Autodesk Fusion 360 part; units mm, degrees
note: some values were not read from the file. Set by a fixed rule: which sketch regions a step uses.
(part 12 of 59)
  spline S64 degree 5 poles (17.8246, 37.863) (17.8224, 37.8615) (17.8179, 37.8584) (17.8112, 37.8539) (17.8023, 37.8477) (17.7913, 37.8401) (17.7802, 37.8325) (17.7692, 37.8248) (17.7583, 37.8172) (17.7473, 37.8096) (17.7364, 37.8019) (17.7256, 37.7943) (17.7147, 37.7867) (17.7039, 37.7791) (17.6932, 37.7715) (17.6825, 37.7639) (17.6718, 37.7563) (17.6611, 37.7487) (17.6505, 37.7411) (17.6399, 37.7335) (17.6294, 37.7259) (17.6189, 37.7184) (17.6084, 37.7108) (17.598, 37.7032) (17.5876, 37.6957) (17.5772, 37.6881) (17.5669, 37.6806) (17.5566, 37.6731) (17.5464, 37.6655) (17.5361, 37.658) (17.526, 37.6505) (17.5158, 37.643) (17.5057, 37.6355) (17.4956, 37.628) (17.4856, 37.6205) (17.4756, 37.613) (17.4657, 37.6055) (17.4557, 37.5981) (17.4458, 37.5906) (17.436, 37.5832) (17.4262, 37.5757) (17.4164, 37.5683) (17.4067, 37.5609) (17.397, 37.5534) (17.3873, 37.546) (17.3777, 37.5386) (17.3681, 37.5312) (17.3585, 37.5238) (17.349, 37.5165) (17.3395, 37.5091) (17.3301, 37.5017) (17.3207, 37.4944) (17.3113, 37.4871) (17.302, 37.4797) (17.2927, 37.4724) (17.2835, 37.4651) (17.2743, 37.4578) (17.2651, 37.4505) (17.2559, 37.4432) (17.2469, 37.436) (17.2378, 37.4287) (17.2288, 37.4215) (17.2198, 37.4142) (17.2108, 37.407) (17.2019, 37.3998) (17.1931, 37.3926) (17.1842, 37.3854) (17.1754, 37.3782) (17.1667, 37.3711) (17.158, 37.3639) (17.1493, 37.3568) (17.1407, 37.3496) (17.1321, 37.3425) (17.1235, 37.3354) (17.115, 37.3283) (17.1065, 37.3212) (17.0981, 37.3142) (17.0897, 37.3071) (17.0813, 37.3001) (17.073, 37.2931) (17.0647, 37.2861) (17.0565, 37.2791) (17.0483, 37.2721) (17.0401, 37.2651) (17.032, 37.2582) (17.0239, 37.2512) (17.0159, 37.2443) (17.0079, 37.2374) (16.9999, 37.2305) (16.992, 37.2236) (16.9841, 37.2168) (16.9763, 37.2099) (16.9685, 37.2031) (16.9607, 37.1963) (16.953, 37.1895) (16.9453, 37.1827) (16.9377, 37.1759) (16.9301, 37.1692) (16.9225, 37.1625) (16.915, 37.1558) (16.9075, 37.1491) (16.9001, 37.1424) (16.8927, 37.1357) (16.8854, 37.1291) (16.8781, 37.1225) (16.8708, 37.1159) (16.8636, 37.1093) (16.8564, 37.1027) (16.8492, 37.0962) (16.8421, 37.0897) (16.8351, 37.0831) (16.8281, 37.0767) (16.8211, 37.0702) (16.8142, 37.0638) (16.8073, 37.0573) (16.8004, 37.0509) (16.7936, 37.0446) (16.7869, 37.0382) (16.7801, 37.0319) (16.7735, 37.0255) (16.7668, 37.0192) (16.7602, 37.013) (16.7537, 37.0067) (16.7472, 37.0005) (16.7407, 36.9943) (16.7343, 36.9881) (16.7279, 36.982) (16.7216, 36.9758) (16.7153, 36.9697) (16.7091, 36.9636) (16.7029, 36.9576) (16.6967, 36.9515) (16.6906, 36.9455) (16.6845, 36.9395) (16.6785, 36.9336) (16.6725, 36.9277) (16.6666, 36.9218) (16.6607, 36.9159) (16.6549, 36.91) (16.6491, 36.9042) (16.6433, 36.8984) (16.6376, 36.8926) (16.6319, 36.8869) (16.6263, 36.8812) (16.6207, 36.8755) (16.6152, 36.8698) (16.6097, 36.8642) (16.6043, 36.8586) (16.5989, 36.853) (16.5935, 36.8475) (16.5882, 36.842) (16.583, 36.8365) (16.5778, 36.8311) (16.5726, 36.8257) (16.5675, 36.8203) (16.5624, 36.8149) (16.5574, 36.8096) (16.5524, 36.8043) (16.5475, 36.7991) (16.5426, 36.7939) (16.5378, 36.7887) (16.533, 36.7835) (16.5282, 36.7784) (16.5236, 36.7733) (16.5189, 36.7683) (16.5143, 36.7633) (16.5098, 36.7583) (16.5053, 36.7534) (16.5008, 36.7485) (16.4964, 36.7436) (16.492, 36.7388) (16.4877, 36.734) (16.4835, 36.7293) (16.4793, 36.7246) (16.4751, 36.7199) (16.471, 36.7153) (16.4669, 36.7107) (16.4629, 36.7062) (16.459, 36.7017) (16.455, 36.6972) (16.4512, 36.6928) (16.4474, 36.6884) (16.4436, 36.6841) (16.4399, 36.6798) (16.4362, 36.6755) (16.4326, 36.6713) (16.4291, 36.6672) (16.4256, 36.6631) (16.4221, 36.659) (16.4187, 36.655) (16.4153, 36.651) (16.412, 36.6471) (16.4088, 36.6432) (16.4056, 36.6394) (16.4024, 36.6356) (16.3994, 36.6319) (16.3963, 36.6283) (16.3933, 36.6246) (16.3904, 36.6211) (16.3875, 36.6176) (16.3847, 36.6141) (16.3819, 36.6107) (16.3792, 36.6073) (16.3766, 36.604) (16.374, 36.6008) (16.3714, 36.5976) (16.3689, 36.5945) (16.3665, 36.5914) (16.3641, 36.5884) (16.3618, 36.5855) (16.3595, 36.5826) (16.3573, 36.5798) (16.3551, 36.577) (16.353, 36.5743) (16.351, 36.5717) (16.349, 36.5691) (16.3471, 36.5666) (16.3452, 36.5641) (16.3434, 36.5618) (16.3416, 36.5595) (16.3399, 36.5572) (16.3383, 36.5551) (16.3367, 36.553) (16.3352, 36.551) (16.3338, 36.549) (16.3324, 36.5471) (16.331, 36.5453) (16.3298, 36.5436) (16.3286, 36.542) (16.3274, 36.5404) (16.3263, 36.5389) (16.3253, 36.5375) (16.3244, 36.5362) (16.3235, 36.535) (16.3227, 36.5338) (16.3219, 36.5327) (16.3212, 36.5317) (16.3206, 36.5309) (16.32, 36.5301) (16.3195, 36.5294) (16.3191, 36.5287) (16.3188, 36.5283) (16.3186, 36.5281) (16.3185, 36.5279) (16.3184, 36.5278) knots -1 -1 -1 -1 -1 -1 -0.99583333 -0.99166667 -0.9875 -0.98333333 -0.97916667 -0.975 -0.97083333 -0.96666667 -0.9625 -0.95833333 -0.95416667 -0.95 -0.94583333 -0.94166667 -0.9375 -0.93333333 -0.92916667 -0.925 -0.92083333 -0.91666667 -0.9125 -0.90833333 -0.90416667 -0.9 -0.89583333 -0.89166667 -0.8875 -0.88333333 -0.87916667 -0.875 -0.87083333 -0.86666667 -0.8625 -0.85833333 -0.85416667 -0.85 -0.84583333 -0.84166667 -0.8375 -0.83333333 -0.82916667 -0.825 -0.82083333 -0.81666667 -0.8125 -0.80833333 -0.80416667 -0.8 -0.79583333 -0.79166667 -0.7875 -0.78333333 -0.77916667 -0.775 -0.77083333 -0.76666667 -0.7625 -0.75833333 -0.75416667 -0.75 -0.74583333 -0.74166667 -0.7375 -0.73333333 -0.72916667 -0.725 -0.72083333 -0.71666667 -0.7125 -0.70833333 -0.70416667 -0.7 -0.69583333 -0.69166667 -0.6875 -0.68333333 -0.67916667 -0.675 -0.67083333 -0.66666667 -0.6625 -0.65833333 -0.65416667 -0.65 -0.64583333 -0.64166667 -0.6375 -0.63333333 -0.62916667 -0.625 -0.62083333 -0.61666667 -0.6125 -0.60833333 -0.60416667 -0.6 -0.59583333 -0.59166667 -0.5875 -0.58333333 -0.57916667 -0.575 -0.57083333 -0.56666667 -0.5625 -0.55833333 -0.55416667 -0.55 -0.54583333 -0.54166667 -0.5375 -0.53333333 -0.52916667 -0.525 -0.52083333 -0.51666667 -0.5125 -0.50833333 -0.50416667 -0.5 -0.49583333 -0.49166667 -0.4875 -0.48333333 -0.47916667 -0.475 -0.47083333 -0.46666667 -0.4625 -0.45833333 -0.45416667 -0.45 -0.44583333 -0.44166667 -0.4375 -0.43333333 -0.42916667 -0.425 -0.42083333 -0.41666667 -0.4125 -0.40833333 -0.40416667 -0.4 -0.39583333 -0.39166667 -0.3875 -0.38333333 -0.37916667 -0.375 -0.37083333 -0.36666667 -0.3625 -0.35833333 -0.35416667 -0.35 -0.34583333 -0.34166667 -0.3375 -0.33333333 -0.32916667 -0.325 -0.32083333 -0.31666667 -0.3125 -0.30833333 -0.30416667 -0.3 -0.29583333 -0.29166667 -0.2875 -0.28333333 -0.27916667 -0.275 -0.27083333 -0.26666667 -0.2625 -0.25833333 -0.25416667 -0.25 -0.24583333 -0.24166667 -0.2375 -0.23333333 -0.22916667 -0.225 -0.22083333 -0.21666667 -0.2125 -0.20833333 -0.20416667 -0.2 -0.19583333 -0.19166667 -0.1875 -0.18333333 -0.17916667 -0.175 -0.17083333 -0.16666667 -0.1625 -0.15833333 -0.15416667 -0.15 -0.14583333 -0.14166667 -0.1375 -0.13333333 -0.12916667 -0.125 -0.12083333 -0.11666667 -0.1125 -0.10833333 -0.10416667 -0.1 -0.09583333 -0.09166667 -0.0875 -0.08333333 -0.07916667 -0.075 -0.07083333 -0.06666667 -0.0625 -0.05833333 -0.05416667 -0.05 -0.04583333 -0.04166667 -0.0375 -0.03333333 -0.02916667 -0.025 -0.02083333 -0.01666667 -0.0125 -0.00833333 -0.00416667 0 0 0 0 0 0
  line L140 (26.8955, 1.5338) -> (26.8948, 1.5341)
  line L141 (12.6495, -13.6461) -> (12.6491, -13.6453)
  line L142 (-28.9671, 14.6182) -> (-28.6734, 14.5967)
  line L143 (20.9575, 32.61) -> (20.9569, 32.6094)
  line L144 (21.9649, 31.0501) -> (22.1898, 31.2401)
  line L145 (-28.2039, 5.5632) -> (-27.918, 5.6335)
  spline S65 degree 5 poles (18.7406, -9.6904) (18.7407, -9.6905) (18.7408, -9.6907) (18.741, -9.6909) (18.7414, -9.6913) (18.7419, -9.6919) (18.7424, -9.6925) (18.7431, -9.6933) (18.7438, -9.6941) (18.7446, -9.695) (18.7455, -9.696) (18.7464, -9.697) (18.7474, -9.6982) (18.7485, -9.6994) (18.7497, -9.7007) (18.7509, -9.702) (18.7522, -9.7035) (18.7536, -9.705) (18.755, -9.7066) (18.7565, -9.7082) (18.7581, -9.7099) (18.7597, -9.7117) (18.7615, -9.7136) (18.7632, -9.7155) (18.7651, -9.7175) (18.767, -9.7195) (18.769, -9.7216) (18.771, -9.7238) (18.7732, -9.726) (18.7753, -9.7283) (18.7776, -9.7307) (18.7799, -9.7331) (18.7823, -9.7355) (18.7847, -9.738) (18.7872, -9.7406) (18.7897, -9.7433) (18.7924, -9.7459) (18.7951, -9.7487) (18.7978, -9.7515) (18.8006, -9.7543) (18.8035, -9.7572) (18.8064, -9.7602) (18.8094, -9.7632) (18.8124, -9.7662) (18.8156, -9.7693) (18.8187, -9.7725) (18.822, -9.7757) (18.8252, -9.7789) (18.8286, -9.7822) (18.832, -9.7855) (18.8355, -9.7889) (18.839, -9.7923) (18.8426, -9.7958) (18.8462, -9.7993) (18.8499, -9.8029) (18.8536, -9.8065) (18.8574, -9.8101) (18.8613, -9.8138) (18.8652, -9.8175) (18.8692, -9.8212) (18.8732, -9.825) (18.8773, -9.8289) (18.8814, -9.8328) (18.8856, -9.8367) (18.8899, -9.8406) (18.8942, -9.8446) (18.8986, -9.8486) (18.903, -9.8527) (18.9074, -9.8568) (18.9119, -9.8609) (18.9165, -9.8651) (18.9211, -9.8693) (18.9258, -9.8736) (18.9306, -9.8778) (18.9353, -9.8821) (18.9402, -9.8865) (18.9451, -9.8909) (18.95, -9.8953) (18.955, -9.8997) (18.96, -9.9042) (18.9651, -9.9087) (18.9703, -9.9132) (18.9755, -9.9177) (18.9807, -9.9223) (18.986, -9.927) (18.9914, -9.9316) (18.9968, -9.9363) (19.0022, -9.941) (19.0077, -9.9457) (19.0133, -9.9505) (19.0189, -9.9553) (19.0246, -9.9601) (19.0303, -9.9649) (19.036, -9.9698) (19.0418, -9.9747) (19.0477, -9.9796) (19.0536, -9.9846) (19.0595, -9.9895) (19.0655, -9.9945) (19.0715, -9.9996) (19.0776, -10.0046) (19.0838, -10.0097) (19.09, -10.0148) (19.0962, -10.0199) (19.1025, -10.025) (19.1088, -10.0302) (19.1152, -10.0354) (19.1216, -10.0406) (19.1281, -10.0458) (19.1346, -10.0511) (19.1412, -10.0564) (19.1478, -10.0617) (19.1544, -10.067) (19.1611, -10.0723) (19.1679, -10.0777) (19.1747, -10.083) (19.1815, -10.0884) (19.1884, -10.0939) (19.1954, -10.0993) (19.2024, -10.1048) (19.2094, -10.1102) (19.2165, -10.1157) (19.2236, -10.1212) (19.2307, -10.1268) (19.2379, -10.1323) (19.2452, -10.1379) (19.2525, -10.1435) (19.2598, -10.1491) (19.2672, -10.1547) (19.2747, -10.1603) (19.2821, -10.166) (19.2897, -10.1716) (19.2972, -10.1773) (19.3048, -10.183) (19.3125, -10.1887) (19.3202, -10.1945) (19.3279, -10.2002) (19.3357, -10.206) (19.3436, -10.2118) (19.3514, -10.2175) (19.3593, -10.2233) (19.3673, -10.2292) (19.3753, -10.235) (19.3834, -10.2408) (19.3914, -10.2467) (19.3996, -10.2526) (19.4078, -10.2585) (19.416, -10.2644) (19.4242, -10.2703) (19.4325, -10.2762) (19.4409, -10.2822) (19.4493, -10.2881) (19.4577, -10.2941) (19.4662, -10.3) (19.4747, -10.306) (19.4832, -10.312) (19.4918, -10.318) (19.5005, -10.3241) (19.5091, -10.3301) (19.5179, -10.3361) (19.5266, -10.3422) (19.5354, -10.3483) (19.5443, -10.3543) (19.5532, -10.3604) (19.5621, -10.3665) (19.5711, -10.3726) (19.5801, -10.3787) (19.5891, -10.3849) (19.5982, -10.391) (19.6073, -10.3971) (19.6165, -10.4033) (19.6257, -10.4095) (19.635, -10.4156) (19.6443, -10.4218) (19.6536, -10.428) (19.663, -10.4342) (19.6724, -10.4404) (19.6818, -10.4466) (19.6913, -10.4528) (19.7009, -10.4591) (19.7104, -10.4653) (19.72, -10.4715) (19.7297, -10.4778) (19.7394, -10.484) (19.7491, -10.4903) (19.7589, -10.4966) (19.7687, -10.5029) (19.7785, -10.5091) (19.7884, -10.5154) (19.7984, -10.5217) (19.8083, -10.528) (19.8183, -10.5343) (19.8284, -10.5406) (19.8384, -10.547) (19.8486, -10.5533) (19.8587, -10.5596) (19.8689, -10.566) (19.8791, -10.5723) (19.8894, -10.5786) (19.8997, -10.585) (19.9101, -10.5914) (19.9205, -10.5977) (19.9309, -10.6041) (19.9413, -10.6104) (19.9518, -10.6168) (19.9624, -10.6232) (19.973, -10.6296) (19.9836, -10.636) (19.9942, -10.6423) (20.0049, -10.6487) (20.0156, -10.6551) (20.0264, -10.6615) (20.0372, -10.6679) (20.048, -10.6743) (20.0589, -10.6807) (20.0698, -10.6872) (20.0808, -10.6936) (20.0917, -10.7) (20.1028, -10.7064) (20.1138, -10.7128) (20.1249, -10.7193) (20.136, -10.7257) (20.1472, -10.7321) (20.1584, -10.7385) (20.1697, -10.745) (20.1809, -10.7514) (20.1922, -10.7578) (20.2036, -10.7643) (20.215, -10.7707) (20.2264, -10.7771) (20.2379, -10.7836) (20.2493, -10.79) (20.2609, -10.7965) (20.2724, -10.8029) (20.284, -10.8094) (20.2957, -10.8158) (20.3073, -10.8222) (20.319, -10.8287) (20.3308, -10.8351) (20.3426, -10.8416) (20.3544, -10.848) (20.3639, -10.8532) (20.371, -10.8571) (20.3757, -10.8596) (20.3781, -10.8609) knots 0 0 0 0 0 0 0.00416667 0.00833333 0.0125 0.01666667 0.02083333 0.025 0.02916667 0.03333333 0.0375 0.04166667 0.04583333 0.05 0.05416667 0.05833333 0.0625 0.06666667 0.07083333 0.075 0.07916667 0.08333333 0.0875 0.09166667 0.09583333 0.1 0.10416667 0.10833333 0.1125 0.11666667 0.12083333 0.125 0.12916667 0.13333333 0.1375 0.14166667 0.14583333 0.15 0.15416667 0.15833333 0.1625 0.16666667 0.17083333 0.175 0.17916667 0.18333333 0.1875 0.19166667 0.19583333 0.2 0.20416667 0.20833333 0.2125 0.21666667 0.22083333 0.225 0.22916667 0.23333333 0.2375 0.24166667 0.24583333 0.25 0.25416667 0.25833333 0.2625 0.26666667 0.27083333 0.275 0.27916667 0.28333333 0.2875 0.29166667 0.29583333 0.3 0.30416667 0.30833333 0.3125 0.31666667 0.32083333 0.325 0.32916667 0.33333333 0.3375 0.34166667 0.34583333 0.35 0.35416667 0.35833333 0.3625 0.36666667 0.37083333 0.375 0.37916667 0.38333333 0.3875 0.39166667 0.39583333 0.4 0.40416667 0.40833333 0.4125 0.41666667 0.42083333 0.425 0.42916667 0.43333333 0.4375 0.44166667 0.44583333 0.45 0.45416667 0.45833333 0.4625 0.46666667 0.47083333 0.475 0.47916667 0.48333333 0.4875 0.49166667 0.49583333 0.5 0.50416667 0.50833333 0.5125 0.51666667 0.52083333 0.525 0.52916667 0.53333333 0.5375 0.54166667 0.54583333 0.55 0.55416667 0.55833333 0.5625 0.56666667 0.57083333 0.575 0.57916667 0.58333333 0.5875 0.59166667 0.59583333 0.6 0.60416667 0.60833333 0.6125 0.61666667 0.62083333 0.625 0.62916667 0.63333333 0.6375 0.64166667 0.64583333 0.65 0.65416667 0.65833333 0.6625 0.66666667 0.67083333 0.675 0.67916667 0.68333333 0.6875 0.69166667 0.69583333 0.7 0.70416667 0.70833333 0.7125 0.71666667 0.72083333 0.725 0.72916667 0.73333333 0.7375 0.74166667 0.74583333 0.75 0.75416667 0.75833333 0.7625 0.76666667 0.77083333 0.775 0.77916667 0.78333333 0.7875 0.79166667 0.79583333 0.8 0.80416667 0.80833333 0.8125 0.81666667 0.82083333 0.825 0.82916667 0.83333333 0.8375 0.84166667 0.84583333 0.85 0.85416667 0.85833333 0.8625 0.86666667 0.87083333 0.875 0.87916667 0.88333333 0.8875 0.89166667 0.89583333 0.9 0.90416667 0.90833333 0.9125 0.91666667 0.92083333 0.925 0.92916667 0.93333333 0.9375 0.94166667 0.94583333 0.95 0.95416667 0.95833333 0.9625 0.96666667 0.97083333 0.975 0.97916667 0.98333333 0.9875 0.99166667 0.99583333 1 1 1 1 1 1
  arc A72 (-13.0527, -15.6181) -> (-12.1618, -16.0147) centre (0, 12.5) ccw
  arc A73 (-13.578, -12.8417) -> (-12.5209, -13.3803) centre (0, 12.5) ccw
  arc A74 (20.3781, -10.8609) -> (21.1029, -10.2084) centre (0, 12.5) ccw
  spline S66 degree 5 poles (-30.8773, 15.255) (-30.8749, 15.2539) (-30.87, 15.2515) (-30.8627, 15.248) (-30.853, 15.2434) (-30.8408, 15.2376) (-30.8287, 15.2319) (-30.8165, 15.2262) (-30.8044, 15.2205) (-30.7924, 15.2149) (-30.7803, 15.2092) (-30.7683, 15.2036) (-30.7563, 15.1981) (-30.7443, 15.1925) (-30.7323, 15.187) (-30.7204, 15.1815) (-30.7085, 15.1761) (-30.6966, 15.1707) (-30.6847, 15.1653) (-30.6728, 15.1599) (-30.661, 15.1545) (-30.6492, 15.1492) (-30.6374, 15.1439) (-30.6256, 15.1387) (-30.6139, 15.1335) (-30.6022, 15.1283) (-30.5905, 15.1231) (-30.5788, 15.1179) (-30.5672, 15.1128) (-30.5555, 15.1077) (-30.5439, 15.1027) (-30.5324, 15.0977) (-30.5208, 15.0927) (-30.5093, 15.0877) (-30.4978, 15.0827) (-30.4863, 15.0778) (-30.4749, 15.0729) (-30.4634, 15.0681) (-30.452, 15.0632) (-30.4407, 15.0584) (-30.4293, 15.0537) (-30.418, 15.0489) (-30.4067, 15.0442) (-30.3954, 15.0395) (-30.3841, 15.0348) (-30.3729, 15.0302) (-30.3617, 15.0256) (-30.3506, 15.021) (-30.3394, 15.0165) (-30.3283, 15.0119) (-30.3172, 15.0074) (-30.3061, 15.003) (-30.2951, 14.9985) (-30.2841, 14.9941) (-30.2731, 14.9897) (-30.2621, 14.9854) (-30.2512, 14.981) (-30.2403, 14.9767) (-30.2294, 14.9725) (-30.2186, 14.9682) (-30.2078, 14.964) (-30.197, 14.9598) (-30.1862, 14.9557) (-30.1755, 14.9515) (-30.1648, 14.9474) (-30.1541, 14.9433) (-30.1435, 14.9393) (-30.1329, 14.9353) (-30.1223, 14.9313) (-30.1118, 14.9273) (-30.1012, 14.9234) (-30.0907, 14.9194) (-30.0803, 14.9156) (-30.0699, 14.9117) (-30.0595, 14.9079) (-30.0491, 14.9041) (-30.0388, 14.9003) (-30.0284, 14.8965) (-30.0182, 14.8928) (-30.0079, 14.8891) (-29.9977, 14.8855) (-29.9875, 14.8818) (-29.9774, 14.8782) (-29.9673, 14.8746) (-29.9572, 14.8711) (-29.9471, 14.8675) (-29.9371, 14.864) (-29.9271, 14.8606) (-29.9172, 14.8571) (-29.9073, 14.8537) (-29.8974, 14.8503) (-29.8875, 14.8469) (-29.8777, 14.8436) (-29.868, 14.8403) (-29.8582, 14.837) (-29.8485, 14.8337) (-29.8388, 14.8305) (-29.8292, 14.8273) (-29.8196, 14.8241) (-29.81, 14.821) (-29.8005, 14.8178) (-29.791, 14.8147) (-29.7815, 14.8117) (-29.7721, 14.8086) (-29.7627, 14.8056) (-29.7534, 14.8026) (-29.7441, 14.7996) (-29.7348, 14.7967) (-29.7255, 14.7938) (-29.7163, 14.7909) (-29.7072, 14.788) (-29.6981, 14.7852) (-29.689, 14.7824) (-29.6799, 14.7796) (-29.6709, 14.7769) (-29.6619, 14.7741) (-29.653, 14.7714) (-29.6441, 14.7688) (-29.6353, 14.7661) (-29.6265, 14.7635) (-29.6177, 14.7609) (-29.609, 14.7583) (-29.6003, 14.7558) (-29.5917, 14.7533) (-29.583, 14.7508) (-29.5745, 14.7483) (-29.566, 14.7458) (-29.5575, 14.7434) (-29.5491, 14.741) (-29.5407, 14.7387) (-29.5323, 14.7363) (-29.524, 14.734) (-29.5158, 14.7317) (-29.5075, 14.7295) (-29.4994, 14.7272) (-29.4912, 14.725) (-29.4832, 14.7228) (-29.4751, 14.7207) (-29.4671, 14.7185) (-29.4592, 14.7164) (-29.4513, 14.7143) (-29.4434, 14.7123) (-29.4356, 14.7102) (-29.4279, 14.7082) (-29.4202, 14.7062) (-29.4125, 14.7043) (-29.4049, 14.7023) (-29.3973, 14.7004) (-29.3898, 14.6985) (-29.3823, 14.6967) (-29.3749, 14.6948) (-29.3675, 14.693) (-29.3602, 14.6912) (-29.3529, 14.6895) (-29.3457, 14.6877) (-29.3386, 14.686) (-29.3314, 14.6843) (-29.3244, 14.6827) (-29.3174, 14.681) (-29.3104, 14.6794) (-29.3035, 14.6778) (-29.2967, 14.6762) (-29.2899, 14.6747) (-29.2831, 14.6731) (-29.2764, 14.6716) (-29.2698, 14.6702) (-29.2632, 14.6687) (-29.2567, 14.6673) (-29.2502, 14.6659) (-29.2438, 14.6645) (-29.2374, 14.6631) (-29.2311, 14.6618) (-29.2249, 14.6605) (-29.2187, 14.6592) (-29.2126, 14.6579) (-29.2065, 14.6567) (-29.2005, 14.6554) (-29.1946, 14.6542) (-29.1887, 14.653) (-29.1829, 14.6519) (-29.1771, 14.6507) (-29.1714, 14.6496) (-29.1658, 14.6485) (-29.1602, 14.6475) (-29.1547, 14.6464) (-29.1493, 14.6454) (-29.1439, 14.6444) (-29.1386, 14.6434) (-29.1334, 14.6424) (-29.1282, 14.6415) (-29.1231, 14.6406) (-29.118, 14.6397) (-29.1131, 14.6388) (-29.1081, 14.638) (-29.1033, 14.6371) (-29.0985, 14.6363) (-29.0938, 14.6355) (-29.0892, 14.6347) (-29.0847, 14.634) (-29.0802, 14.6332) (-29.0758, 14.6325) (-29.0714, 14.6318) (-29.0672, 14.6312) (-29.063, 14.6305) (-29.0589, 14.6299) (-29.0549, 14.6292) (-29.0509, 14.6286) (-29.047, 14.6281) (-29.0432, 14.6275) (-29.0395, 14.627) (-29.0359, 14.6264) (-29.0323, 14.6259) (-29.0289, 14.6254) (-29.0255, 14.625) (-29.0222, 14.6245) (-29.0189, 14.6241) (-29.0158, 14.6237) (-29.0128, 14.6233) (-29.0098, 14.6229) (-29.0069, 14.6225) (-29.0041, 14.6222) (-29.0015, 14.6219) (-28.9989, 14.6215) (-28.9963, 14.6212) (-28.9939, 14.621) (-28.9916, 14.6207) (-28.9894, 14.6204) (-28.9873, 14.6202) (-28.9852, 14.62) (-28.9833, 14.6198) (-28.9815, 14.6196) (-28.9798, 14.6194) (-28.9781, 14.6192) (-28.9766, 14.6191) (-28.9752, 14.6189) (-28.9739, 14.6188) (-28.9727, 14.6187) (-28.9716, 14.6186) (-28.9706, 14.6185) (-28.9698, 14.6184) (-28.969, 14.6184) (-28.9685, 14.6183) (-28.9682, 14.6183) (-28.968, 14.6183) (-28.9679, 14.6183) knots -1 -1 -1 -1 -1 -1 -0.99583333 -0.99166667 -0.9875 -0.98333333 -0.97916667 -0.975 -0.97083333 -0.96666667 -0.9625 -0.95833333 -0.95416667 -0.95 -0.94583333 -0.94166667 -0.9375 -0.93333333 -0.92916667 -0.925 -0.92083333 -0.91666667 -0.9125 -0.90833333 -0.90416667 -0.9 -0.89583333 -0.89166667 -0.8875 -0.88333333 -0.87916667 -0.875 -0.87083333 -0.86666667 -0.8625 -0.85833333 -0.85416667 -0.85 -0.84583333 -0.84166667 -0.8375 -0.83333333 -0.82916667 -0.825 -0.82083333 -0.81666667 -0.8125 -0.80833333 -0.80416667 -0.8 -0.79583333 -0.79166667 -0.7875 -0.78333333 -0.77916667 -0.775 -0.77083333 -0.76666667 -0.7625 -0.75833333 -0.75416667 -0.75 -0.74583333 -0.74166667 -0.7375 -0.73333333 -0.72916667 -0.725 -0.72083333 -0.71666667 -0.7125 -0.70833333 -0.70416667 -0.7 -0.69583333 -0.69166667 -0.6875 -0.68333333 -0.67916667 -0.675 -0.67083333 -0.66666667 -0.6625 -0.65833333 -0.65416667 -0.65 -0.64583333 -0.64166667 -0.6375 -0.63333333 -0.62916667 -0.625 -0.62083333 -0.61666667 -0.6125 -0.60833333 -0.60416667 -0.6 -0.59583333 -0.59166667 -0.5875 -0.58333333 -0.57916667 -0.575 -0.57083333 -0.56666667 -0.5625 -0.55833333 -0.55416667 -0.55 -0.54583333 -0.54166667 -0.5375 -0.53333333 -0.52916667 -0.525 -0.52083333 -0.51666667 -0.5125 -0.50833333 -0.50416667 -0.5 -0.49583333 -0.49166667 -0.4875 -0.48333333 -0.47916667 -0.475 -0.47083333 -0.46666667 -0.4625 -0.45833333 -0.45416667 -0.45 -0.44583333 -0.44166667 -0.4375 -0.43333333 -0.42916667 -0.425 -0.42083333 -0.41666667 -0.4125 -0.40833333 -0.40416667 -0.4 -0.39583333 -0.39166667 -0.3875 -0.38333333 -0.37916667 -0.375 -0.37083333 -0.36666667 -0.3625 -0.35833333 -0.35416667 -0.35 -0.34583333 -0.34166667 -0.3375 -0.33333333 -0.32916667 -0.325 -0.32083333 -0.31666667 -0.3125 -0.30833333 -0.30416667 -0.3 -0.29583333 -0.29166667 -0.2875 -0.28333333 -0.27916667 -0.275 -0.27083333 -0.26666667 -0.2625 -0.25833333 -0.25416667 -0.25 -0.24583333 -0.24166667 -0.2375 -0.23333333 -0.22916667 -0.225 -0.22083333 -0.21666667 -0.2125 -0.20833333 -0.20416667 -0.2 -0.19583333 -0.19166667 -0.1875 -0.18333333 -0.17916667 -0.175 -0.17083333 -0.16666667 -0.1625 -0.15833333 -0.15416667 -0.15 -0.14583333 -0.14166667 -0.1375 -0.13333333 -0.12916667 -0.125 -0.12083333 -0.11666667 -0.1125 -0.10833333 -0.10416667 -0.1 -0.09583333 -0.09166667 -0.0875 -0.08333333 -0.07916667 -0.075 -0.07083333 -0.06666667 -0.0625 -0.05833333 -0.05416667 -0.05 -0.04583333 -0.04166667 -0.0375 -0.03333333 -0.02916667 -0.025 -0.02083333 -0.01666667 -0.0125 -0.00833333 -0.00416667 0 0 0 0 0 0
  line L146 (22.9448, 30.3091) -> (22.9441, 30.3086)
  spline S67 degree 5 poles (-28.7753, 16.4508) (-28.7754, 16.4508) (-28.7756, 16.4508) (-28.7759, 16.4509) (-28.7764, 16.4509) (-28.7772, 16.451) (-28.778, 16.4511) (-28.779, 16.4512) (-28.7801, 16.4514) (-28.7813, 16.4515) (-28.7826, 16.4517) (-28.784, 16.4518) (-28.7855, 16.452) (-28.7871, 16.4522) (-28.7889, 16.4523) (-28.7907, 16.4525) (-28.7926, 16.4527) (-28.7946, 16.4529) (-28.7968, 16.4531) (-28.799, 16.4534) (-28.8013, 16.4536) (-28.8037, 16.4538) (-28.8063, 16.454) (-28.8089, 16.4543) (-28.8116, 16.4545) (-28.8144, 16.4547) (-28.8172, 16.455) (-28.8202, 16.4552) (-28.8233, 16.4555) (-28.8264, 16.4557) (-28.8297, 16.4559) (-28.833, 16.4562) (-28.8364, 16.4564) (-28.8399, 16.4567) (-28.8435, 16.4569) (-28.8472, 16.4572) (-28.8509, 16.4574) (-28.8547, 16.4577) (-28.8586, 16.4579) (-28.8626, 16.4581) (-28.8667, 16.4584) (-28.8709, 16.4586) (-28.8751, 16.4588) (-28.8794, 16.459) (-28.8838, 16.4593) (-28.8882, 16.4595) (-28.8928, 16.4597) (-28.8974, 16.4599) (-28.9021, 16.4601) (-28.9068, 16.4603) (-28.9117, 16.4605) (-28.9166, 16.4607) (-28.9215, 16.4609) (-28.9266, 16.461) (-28.9317, 16.4612) (-28.9369, 16.4614) (-28.9422, 16.4615) (-28.9475, 16.4617) (-28.9529, 16.4618) (-28.9584, 16.462) (-28.9639, 16.4621) (-28.9695, 16.4622) (-28.9752, 16.4623) (-28.9809, 16.4624) (-28.9867, 16.4625) (-28.9926, 16.4626) (-28.9985, 16.4627) (-29.0045, 16.4627) (-29.0106, 16.4628) (-29.0167, 16.4629) (-29.0229, 16.4629) (-29.0291, 16.4629) (-29.0355, 16.4629) (-29.0418, 16.463) (-29.0483, 16.463) (-29.0548, 16.4629) (-29.0613, 16.4629) (-29.068, 16.4629) (-29.0746, 16.4628) (-29.0814, 16.4628) (-29.0882, 16.4627) (-29.095, 16.4626) (-29.1019, 16.4626) (-29.1089, 16.4625) (-29.1159, 16.4623) (-29.123, 16.4622) (-29.1302, 16.4621) (-29.1374, 16.4619) (-29.1446, 16.4618) (-29.1519, 16.4616) (-29.1593, 16.4614) (-29.1667, 16.4612) (-29.1742, 16.461) (-29.1817, 16.4607) (-29.1893, 16.4605) (-29.197, 16.4603) (-29.2047, 16.46) (-29.2124, 16.4597) (-29.2202, 16.4594) (-29.2281, 16.4591) (-29.236, 16.4588) (-29.2439, 16.4584) (-29.2519, 16.4581) (-29.26, 16.4577) (-29.2681, 16.4573) (-29.2763, 16.4569) (-29.2845, 16.4565) (-29.2927, 16.4561) (-29.301, 16.4556) (-29.3094, 16.4552) (-29.3178, 16.4547) (-29.3263, 16.4542) (-29.3348, 16.4537) (-29.3433, 16.4532) (-29.3519, 16.4526) (-29.3606, 16.4521) (-29.3693, 16.4515) (-29.378, 16.4509) (-29.3868, 16.4503) (-29.3957, 16.4497) (-29.4045, 16.4491) (-29.4135, 16.4484) (-29.4225, 16.4478) (-29.4315, 16.4471) (-29.4406, 16.4464) (-29.4497, 16.4457) (-29.4588, 16.4449) (-29.468, 16.4442) (-29.4773, 16.4434) (-29.4866, 16.4426) (-29.4959, 16.4418) (-29.5053, 16.441) (-29.5147, 16.4402) (-29.5242, 16.4393) (-29.5337, 16.4384) (-29.5433, 16.4375) (-29.5529, 16.4366) (-29.5625, 16.4357) (-29.5722, 16.4348) (-29.5819, 16.4338) (-29.5917, 16.4328) (-29.6015, 16.4318) (-29.6113, 16.4308) (-29.6212, 16.4297) (-29.6312, 16.4287) (-29.6411, 16.4276) (-29.6512, 16.4265) (-29.6612, 16.4254) (-29.6713, 16.4243) (-29.6814, 16.4231) (-29.6916, 16.422) (-29.7018, 16.4208) (-29.7121, 16.4196) (-29.7224, 16.4183) (-29.7327, 16.4171) (-29.7431, 16.4158) (-29.7535, 16.4145) (-29.764, 16.4132) (-29.7744, 16.4119) (-29.785, 16.4106) (-29.7955, 16.4092) (-29.8061, 16.4078) (-29.8168, 16.4064) (-29.8274, 16.405) (-29.8382, 16.4035) (-29.8489, 16.4021) (-29.8597, 16.4006) (-29.8705, 16.3991) (-29.8814, 16.3976) (-29.8923, 16.396) (-29.9032, 16.3945) (-29.9142, 16.3929) (-29.9252, 16.3913) (-29.9362, 16.3896) (-29.9473, 16.388) (-29.9584, 16.3863) (-29.9696, 16.3846) (-29.9807, 16.3829) (-29.992, 16.3812) (-30.0032, 16.3795) (-30.0145, 16.3777) (-30.0258, 16.3759) (-30.0372, 16.3741) (-30.0486, 16.3722) (-30.06, 16.3704) (-30.0714, 16.3685) (-30.0829, 16.3666) (-30.0944, 16.3647) (-30.106, 16.3628) (-30.1176, 16.3608) (-30.1292, 16.3588) (-30.1409, 16.3568) (-30.1525, 16.3548) (-30.1643, 16.3527) (-30.176, 16.3507) (-30.1878, 16.3486) (-30.1996, 16.3464) (-30.2115, 16.3443) (-30.2233, 16.3422) (-30.2353, 16.34) (-30.2472, 16.3378) (-30.2592, 16.3356) (-30.2712, 16.3333) (-30.2832, 16.331) (-30.2953, 16.3288) (-30.3074, 16.3264) (-30.3195, 16.3241) (-30.3317, 16.3217) (-30.3439, 16.3194) (-30.3561, 16.317) (-30.3683, 16.3145) (-30.3806, 16.3121) (-30.3929, 16.3096) (-30.4053, 16.3071) (-30.4176, 16.3046) (-30.43, 16.3021) (-30.4424, 16.2995) (-30.4549, 16.297) (-30.4674, 16.2943) (-30.4799, 16.2917) (-30.4924, 16.2891) (-30.505, 16.2864) (-30.5176, 16.2837) (-30.5302, 16.281) (-30.5429, 16.2782) (-30.5556, 16.2755) (-30.5683, 16.2727) (-30.581, 16.2699) (-30.5938, 16.267) (-30.6066, 16.2642) (-30.6194, 16.2613) (-30.6323, 16.2584) (-30.6451, 16.2555) (-30.658, 16.2525) (-30.671, 16.2496) (-30.6839, 16.2466) (-30.6969, 16.2435) (-30.7099, 16.2405) (-30.723, 16.2374) (-30.736, 16.2343) (-30.7491, 16.2312) (-30.7596, 16.2287) (-30.7675, 16.2268) (-30.7728, 16.2256) (-30.7754, 16.2249) knots 0 0 0 0 0 0 0.00416667 0.00833333 0.0125 0.01666667 0.02083333 0.025 0.02916667 0.03333333 0.0375 0.04166667 0.04583333 0.05 0.05416667 0.05833333 0.0625 0.06666667 0.07083333 0.075 0.07916667 0.08333333 0.0875 0.09166667 0.09583333 0.1 0.10416667 0.10833333 0.1125 0.11666667 0.12083333 0.125 0.12916667 0.13333333 0.1375 0.14166667 0.14583333 0.15 0.15416667 0.15833333 0.1625 0.16666667 0.17083333 0.175 0.17916667 0.18333333 0.1875 0.19166667 0.19583333 0.2 0.20416667 0.20833333 0.2125 0.21666667 0.22083333 0.225 0.22916667 0.23333333 0.2375 0.24166667 0.24583333 0.25 0.25416667 0.25833333 0.2625 0.26666667 0.27083333 0.275 0.27916667 0.28333333 0.2875 0.29166667 0.29583333 0.3 0.30416667 0.30833333 0.3125 0.31666667 0.32083333 0.325 0.32916667 0.33333333 0.3375 0.34166667 0.34583333 0.35 0.35416667 0.35833333 0.3625 0.36666667 0.37083333 0.375 0.37916667 0.38333333 0.3875 0.39166667 0.39583333 0.4 0.40416667 0.40833333 0.4125 0.41666667 0.42083333 0.425 0.42916667 0.43333333 0.4375 0.44166667 0.44583333 0.45 0.45416667 0.45833333 0.4625 0.46666667 0.47083333 0.475 0.47916667 0.48333333 0.4875 0.49166667 0.49583333 0.5 0.50416667 0.50833333 0.5125 0.51666667 0.52083333 0.525 0.52916667 0.53333333 0.5375 0.54166667 0.54583333 0.55 0.55416667 0.55833333 0.5625 0.56666667 0.57083333 0.575 0.57916667 0.58333333 0.5875 0.59166667 0.59583333 0.6 0.60416667 0.60833333 0.6125 0.61666667 0.62083333 0.625 0.62916667 0.63333333 0.6375 0.64166667 0.64583333 0.65 0.65416667 0.65833333 0.6625 0.66666667 0.67083333 0.675 0.67916667 0.68333333 0.6875 0.69166667 0.69583333 0.7 0.70416667 0.70833333 0.7125 0.71666667 0.72083333 0.725 0.72916667 0.73333333 0.7375 0.74166667 0.74583333 0.75 0.75416667 0.75833333 0.7625 0.76666667 0.77083333 0.775 0.77916667 0.78333333 0.7875 0.79166667 0.79583333 0.8 0.80416667 0.80833333 0.8125 0.81666667 0.82083333 0.825 0.82916667 0.83333333 0.8375 0.84166667 0.84583333 0.85 0.85416667 0.85833333 0.8625 0.86666667 0.87083333 0.875 0.87916667 0.88333333 0.8875 0.89166667 0.89583333 0.9 0.90416667 0.90833333 0.9125 0.91666667 0.92083333 0.925 0.92916667 0.93333333 0.9375 0.94166667 0.94583333 0.95 0.95416667 0.95833333 0.9625 0.96666667 0.97083333 0.975 0.97916667 0.98333333 0.9875 0.99166667 0.99583333 1 1 1 1 1 1
  arc A75 (-30.7754, 16.2249) -> (-30.8773, 15.255) centre (0, 12.5) ccw
  line L147 (-28.2047, 5.563) -> (-28.2039, 5.5632)
  arc A76 (19.9055, -8.2445) -> (20.7445, -7.4055) centre (0, 12.5) ccw
  line L148 (-28.9679, 14.6183) -> (-28.9671, 14.6182)
  arc A77 (-30.9962, 12.9876) -> (-30.9962, 12.0124) centre (0, 12.5) ccw
  spline S68 degree 5 poles (-12.6495, -13.6461) (-12.6495, -13.6462) (-12.6496, -13.6464) (-12.6497, -13.6467) (-12.65, -13.6471) (-12.6503, -13.6478) (-12.6506, -13.6486) (-12.651, -13.6495) (-12.6515, -13.6504) (-12.652, -13.6515) (-12.6526, -13.6527) (-12.6531, -13.654) (-12.6538, -13.6554) (-12.6544, -13.6569) (-12.6551, -13.6585) (-12.6559, -13.6602) (-12.6567, -13.6619) (-12.6575, -13.6638) (-12.6583, -13.6658) (-12.6592, -13.6678) (-12.6602, -13.67) (-12.6611, -13.6722) (-12.6621, -13.6745) (-12.6631, -13.6769) (-12.6642, -13.6794) (-12.6653, -13.682) (-12.6664, -13.6847) (-12.6676, -13.6874) (-12.6687, -13.6903) (-12.6699, -13.6932) (-12.6712, -13.6962) (-12.6724, -13.6993) (-12.6737, -13.7024) (-12.675, -13.7057) (-12.6764, -13.709) (-12.6778, -13.7124) (-12.6791, -13.7159) (-12.6806, -13.7195) (-12.682, -13.7231) (-12.6834, -13.7269) (-12.6849, -13.7307) (-12.6864, -13.7345) (-12.688, -13.7385) (-12.6895, -13.7425) (-12.6911, -13.7466) (-12.6927, -13.7508) (-12.6943, -13.755) (-12.6959, -13.7594) (-12.6975, -13.7638) (-12.6992, -13.7682) (-12.7009, -13.7728) (-12.7026, -13.7774) (-12.7043, -13.782) (-12.706, -13.7868) (-12.7077, -13.7916) (-12.7095, -13.7965) (-12.7113, -13.8015) (-12.7131, -13.8065) (-12.7149, -13.8116) (-12.7167, -13.8167) (-12.7185, -13.822) (-12.7204, -13.8273) (-12.7222, -13.8326) (-12.7241, -13.838) (-12.726, -13.8435) (-12.7279, -13.8491) (-12.7298, -13.8547) (-12.7317, -13.8604) (-12.7336, -13.8661) (-12.7356, -13.8719) (-12.7375, -13.8778) (-12.7395, -13.8837) (-12.7414, -13.8897) (-12.7434, -13.8958) (-12.7454, -13.9019) (-12.7474, -13.9081) (-12.7494, -13.9144) (-12.7514, -13.9207) (-12.7534, -13.927) (-12.7555, -13.9335) (-12.7575, -13.9399) (-12.7596, -13.9465) (-12.7616, -13.9531) (-12.7637, -13.9598) (-12.7657, -13.9665) (-12.7678, -13.9733) (-12.7699, -13.9801) (-12.772, -13.987) (-12.774, -13.9939) (-12.7761, -14.0009) (-12.7782, -14.008) (-12.7803, -14.0151) (-12.7824, -14.0223) (-12.7845, -14.0296) (-12.7867, -14.0368) (-12.7888, -14.0442) (-12.7909, -14.0516) (-12.793, -14.059) (-12.7952, -14.0665) (-12.7973, -14.0741) (-12.7994, -14.0817) (-12.8016, -14.0894) (-12.8037, -14.0971) (-12.8058, -14.1049) (-12.808, -14.1127) (-12.8101, -14.1206) (-12.8123, -14.1286) (-12.8144, -14.1365) (-12.8166, -14.1446) (-12.8187, -14.1527) (-12.8208, -14.1608) (-12.823, -14.169) (-12.8251, -14.1773) (-12.8273, -14.1856) (-12.8294, -14.1939) (-12.8316, -14.2023) (-12.8337, -14.2108) (-12.8359, -14.2193) (-12.838, -14.2278) (-12.8402, -14.2364) (-12.8423, -14.2451) (-12.8445, -14.2537) (-12.8466, -14.2625) (-12.8487, -14.2713) (-12.8509, -14.2801) (-12.853, -14.289) (-12.8551, -14.298) (-12.8573, -14.3069) (-12.8594, -14.316) (-12.8615, -14.3251) (-12.8636, -14.3342) (-12.8658, -14.3434) (-12.8679, -14.3526) (-12.87, -14.3619) (-12.8721, -14.3712) (-12.8742, -14.3806) (-12.8763, -14.39) (-12.8784, -14.3994) (-12.8805, -14.4089) (-12.8826, -14.4185) (-12.8847, -14.4281) (-12.8867, -14.4377) (-12.8888, -14.4474) (-12.8909, -14.4571) (-12.8929, -14.4669) (-12.895, -14.4767) (-12.8971, -14.4866) (-12.8991, -14.4965) (-12.9011, -14.5064) (-12.9032, -14.5164) (-12.9052, -14.5265) (-12.9072, -14.5365) (-12.9093, -14.5467) (-12.9113, -14.5568) (-12.9133, -14.5671) (-12.9153, -14.5773) (-12.9173, -14.5876) (-12.9193, -14.5979) (-12.9213, -14.6083) (-12.9232, -14.6188) (-12.9252, -14.6292) (-12.9272, -14.6397) (-12.9291, -14.6503) (-12.9311, -14.6609) (-12.933, -14.6715) (-12.9349, -14.6822) (-12.9368, -14.6929) (-12.9388, -14.7037) (-12.9407, -14.7145) (-12.9426, -14.7253) (-12.9445, -14.7362) (-12.9463, -14.7471) (-12.9482, -14.7581) (-12.9501, -14.7691) (-12.9519, -14.7801) (-12.9538, -14.7912) (-12.9556, -14.8023) (-12.9574, -14.8135) (-12.9593, -14.8247) (-12.9611, -14.8359) (-12.9629, -14.8472) (-12.9647, -14.8585) (-12.9665, -14.8699) (-12.9682, -14.8813) (-12.97, -14.8927) (-12.9718, -14.9042) (-12.9735, -14.9157) (-12.9752, -14.9273) (-12.977, -14.9388) (-12.9787, -14.9505) (-12.9804, -14.9621) (-12.9821, -14.9738) (-12.9838, -14.9856) (-12.9854, -14.9974) (-12.9871, -15.0092) (-12.9887, -15.021) (-12.9904, -15.0329) (-12.992, -15.0449) (-12.9936, -15.0568) (-12.9952, -15.0688) (-12.9968, -15.0809) (-12.9984, -15.0929) (-13, -15.105) (-13.0016, -15.1172) (-13.0031, -15.1294) (-13.0047, -15.1416) (-13.0062, -15.1539) (-13.0077, -15.1661) (-13.0092, -15.1785) (-13.0107, -15.1908) (-13.0122, -15.2032) (-13.0136, -15.2157) (-13.0151, -15.2281) (-13.0165, -15.2406) (-13.018, -15.2532) (-13.0194, -15.2658) (-13.0208, -15.2784) (-13.0222, -15.291) (-13.0236, -15.3037) (-13.0249, -15.3164) (-13.0263, -15.3291) (-13.0276, -15.3419) (-13.029, -15.3547) (-13.0303, -15.3676) (-13.0316, -15.3805) (-13.0329, -15.3934) (-13.0342, -15.4063) (-13.0354, -15.4193) (-13.0367, -15.4323) (-13.0379, -15.4454) (-13.0391, -15.4585) (-13.0404, -15.4716) (-13.0415, -15.4848) (-13.0427, -15.4979) (-13.0439, -15.5112) (-13.0451, -15.5244) (-13.0462, -15.5377) (-13.0473, -15.551) (-13.0484, -15.5644) (-13.0495, -15.5777) (-13.0506, -15.5911) (-13.0515, -15.6019) (-13.0521, -15.61) (-13.0525, -15.6154) (-13.0527, -15.6181) knots 0 0 0 0 0 0 0.00416667 0.00833333 0.0125 0.01666667 0.02083333 0.025 0.02916667 0.03333333 0.0375 0.04166667 0.04583333 0.05 0.05416667 0.05833333 0.0625 0.06666667 0.07083333 0.075 0.07916667 0.08333333 0.0875 0.09166667 0.09583333 0.1 0.10416667 0.10833333 0.1125 0.11666667 0.12083333 0.125 0.12916667 0.13333333 0.1375 0.14166667 0.14583333 0.15 0.15416667 0.15833333 0.1625 0.16666667 0.17083333 0.175 0.17916667 0.18333333 0.1875 0.19166667 0.19583333 0.2 0.20416667 0.20833333 0.2125 0.21666667 0.22083333 0.225 0.22916667 0.23333333 0.2375 0.24166667 0.24583333 0.25 0.25416667 0.25833333 0.2625 0.26666667 0.27083333 0.275 0.27916667 0.28333333 0.2875 0.29166667 0.29583333 0.3 0.30416667 0.30833333 0.3125 0.31666667 0.32083333 0.325 0.32916667 0.33333333 0.3375 0.34166667 0.34583333 0.35 0.35416667 0.35833333 0.3625 0.36666667 0.37083333 0.375 0.37916667 0.38333333 0.3875 0.39166667 0.39583333 0.4 0.40416667 0.40833333 0.4125 0.41666667 0.42083333 0.425 0.42916667 0.43333333 0.4375 0.44166667 0.44583333 0.45 0.45416667 0.45833333 0.4625 0.46666667 0.47083333 0.475 0.47916667 0.48333333 0.4875 0.49166667 0.49583333 0.5 0.50416667 0.50833333 0.5125 0.51666667 0.52083333 0.525 0.52916667 0.53333333 0.5375 0.54166667 0.54583333 0.55 0.55416667 0.55833333 0.5625 0.56666667 0.57083333 0.575 0.57916667 0.58333333 0.5875 0.59166667 0.59583333 0.6 0.60416667 0.60833333 0.6125 0.61666667 0.62083333 0.625 0.62916667 0.63333333 0.6375 0.64166667 0.64583333 0.65 0.65416667 0.65833333 0.6625 0.66666667 0.67083333 0.675 0.67916667 0.68333333 0.6875 0.69166667 0.69583333 0.7 0.70416667 0.70833333 0.7125 0.71666667 0.72083333 0.725 0.72916667 0.73333333 0.7375 0.74166667 0.74583333 0.75 0.75416667 0.75833333 0.7625 0.76666667 0.77083333 0.775 0.77916667 0.78333333 0.7875 0.79166667 0.79583333 0.8 0.80416667 0.80833333 0.8125 0.81666667 0.82083333 0.825 0.82916667 0.83333333 0.8375 0.84166667 0.84583333 0.85 0.85416667 0.85833333 0.8625 0.86666667 0.87083333 0.875 0.87916667 0.88333333 0.8875 0.89166667 0.89583333 0.9 0.90416667 0.90833333 0.9125 0.91666667 0.92083333 0.925 0.92916667 0.93333333 0.9375 0.94166667 0.94583333 0.95 0.95416667 0.95833333 0.9625 0.96666667 0.97083333 0.975 0.97916667 0.98333333 0.9875 0.99166667 0.99583333 1 1 1 1 1 1
  arc A78 (-10.0421, -16.8284) -> (-9.1146, -17.1298) centre (0, 12.5) ccw
  line L149 (-27.6109, 4.4875) -> (-27.8937, 4.4055)
  arc A79 (-10.8547, -14.1221) -> (-9.7471, -14.5473) centre (0, 12.5) ccw
  arc A80 (-28.6734, 14.5967) -> (-28.7355, 13.4119) centre (0, 12.5) ccw
  line L150 (19.9055, 33.2445) -> (20.1094, 33.4569)
  line L151 (-27.8937, 4.4055) -> (-27.8945, 4.4052)
  spline S69 degree 5 poles (16.3184, -11.5278) (16.3185, -11.5279) (16.3186, -11.5281) (16.3188, -11.5283) (16.3191, -11.5287) (16.3195, -11.5294) (16.32, -11.5301) (16.3206, -11.5309) (16.3212, -11.5317) (16.3219, -11.5327) (16.3227, -11.5338) (16.3235, -11.535) (16.3244, -11.5362) (16.3253, -11.5375) (16.3263, -11.5389) (16.3274, -11.5404) (16.3286, -11.542) (16.3298, -11.5436) (16.331, -11.5453) (16.3324, -11.5471) (16.3338, -11.549) (16.3352, -11.551) (16.3367, -11.553) (16.3383, -11.5551) (16.3399, -11.5572) (16.3416, -11.5595) (16.3434, -11.5618) (16.3452, -11.5641) (16.3471, -11.5666) (16.349, -11.5691) (16.351, -11.5717) (16.353, -11.5743) (16.3551, -11.577) (16.3573, -11.5798) (16.3595, -11.5826) (16.3618, -11.5855) (16.3641, -11.5884) (16.3665, -11.5914) (16.3689, -11.5945) (16.3714, -11.5976) (16.374, -11.6008) (16.3766, -11.604) (16.3792, -11.6073) (16.3819, -11.6107) (16.3847, -11.6141) (16.3875, -11.6176) (16.3904, -11.6211) (16.3933, -11.6246) (16.3963, -11.6283) (16.3994, -11.6319) (16.4024, -11.6356) (16.4056, -11.6394) (16.4088, -11.6432) (16.412, -11.6471) (16.4153, -11.651) (16.4187, -11.655) (16.4221, -11.659) (16.4256, -11.6631) (16.4291, -11.6672) (16.4326, -11.6713) (16.4362, -11.6755) (16.4399, -11.6798) (16.4436, -11.6841) (16.4474, -11.6884) (16.4512, -11.6928) (16.455, -11.6972) (16.459, -11.7017) (16.4629, -11.7062) (16.4669, -11.7107) (16.471, -11.7153) (16.4751, -11.7199) (16.4793, -11.7246) (16.4835, -11.7293) (16.4877, -11.734) (16.492, -11.7388) (16.4964, -11.7436) (16.5008, -11.7485) (16.5053, -11.7534) (16.5098, -11.7583) (16.5143, -11.7633) (16.5189, -11.7683) (16.5236, -11.7733) (16.5282, -11.7784) (16.533, -11.7835) (16.5378, -11.7887) (16.5426, -11.7939) (16.5475, -11.7991) (16.5524, -11.8043) (16.5574, -11.8096) (16.5624, -11.8149) (16.5675, -11.8203) (16.5726, -11.8257) (16.5778, -11.8311) (16.583, -11.8365) (16.5882, -11.842) (16.5935, -11.8475) (16.5989, -11.853) (16.6043, -11.8586) (16.6097, -11.8642) (16.6152, -11.8698) (16.6207, -11.8755) (16.6263, -11.8812) (16.6319, -11.8869) (16.6376, -11.8926) (16.6433, -11.8984) (16.6491, -11.9042) (16.6549, -11.91) (16.6607, -11.9159) (16.6666, -11.9218) (16.6725, -11.9277) (16.6785, -11.9336) (16.6845, -11.9395) (16.6906, -11.9455) (16.6967, -11.9515) (16.7029, -11.9576) (16.7091, -11.9636) (16.7153, -11.9697) (16.7216, -11.9758) (16.7279, -11.982) (16.7343, -11.9881) (16.7407, -11.9943) (16.7472, -12.0005) (16.7537, -12.0067) (16.7602, -12.013) (16.7668, -12.0192) (16.7735, -12.0255) (16.7801, -12.0319) (16.7869, -12.0382) (16.7936, -12.0446) (16.8004, -12.0509) (16.8073, -12.0573) (16.8142, -12.0638) (16.8211, -12.0702) (16.8281, -12.0767) (16.8351, -12.0831) (16.8421, -12.0897) (16.8492, -12.0962) (16.8564, -12.1027) (16.8636, -12.1093) (16.8708, -12.1159) (16.8781, -12.1225) (16.8854, -12.1291) (16.8927, -12.1357) (16.9001, -12.1424) (16.9075, -12.1491) (16.915, -12.1558) (16.9225, -12.1625) (16.9301, -12.1692) (16.9377, -12.1759) (16.9453, -12.1827) (16.953, -12.1895) (16.9607, -12.1963) (16.9685, -12.2031) (16.9763, -12.2099) (16.9841, -12.2168) (16.992, -12.2236) (16.9999, -12.2305) (17.0079, -12.2374) (17.0159, -12.2443) (17.0239, -12.2512) (17.032, -12.2582) (17.0401, -12.2651) (17.0483, -12.2721) (17.0565, -12.2791) (17.0647, -12.2861) (17.073, -12.2931) (17.0813, -12.3001) (17.0897, -12.3071) (17.0981, -12.3142) (17.1065, -12.3212) (17.115, -12.3283) (17.1235, -12.3354) (17.1321, -12.3425) (17.1407, -12.3496) (17.1493, -12.3568) (17.158, -12.3639) (17.1667, -12.3711) (17.1754, -12.3782) (17.1842, -12.3854) (17.1931, -12.3926) (17.2019, -12.3998) (17.2108, -12.407) (17.2198, -12.4142) (17.2288, -12.4215) (17.2378, -12.4287) (17.2469, -12.436) (17.2559, -12.4432) (17.2651, -12.4505) (17.2743, -12.4578) (17.2835, -12.4651) (17.2927, -12.4724) (17.302, -12.4797) (17.3113, -12.4871) (17.3207, -12.4944) (17.3301, -12.5017) (17.3395, -12.5091) (17.349, -12.5165) (17.3585, -12.5238) (17.3681, -12.5312) (17.3777, -12.5386) (17.3873, -12.546) (17.397, -12.5534) (17.4067, -12.5609) (17.4164, -12.5683) (17.4262, -12.5757) (17.436, -12.5832) (17.4458, -12.5906) (17.4557, -12.5981) (17.4657, -12.6055) (17.4756, -12.613) (17.4856, -12.6205) (17.4956, -12.628) (17.5057, -12.6355) (17.5158, -12.643) (17.526, -12.6505) (17.5361, -12.658) (17.5464, -12.6655) (17.5566, -12.6731) (17.5669, -12.6806) (17.5772, -12.6881) (17.5876, -12.6957) (17.598, -12.7032) (17.6084, -12.7108) (17.6189, -12.7184) (17.6294, -12.7259) (17.6399, -12.7335) (17.6505, -12.7411) (17.6611, -12.7487) (17.6718, -12.7563) (17.6825, -12.7639) (17.6932, -12.7715) (17.7039, -12.7791) (17.7147, -12.7867) (17.7256, -12.7943) (17.7364, -12.8019) (17.7473, -12.8096) (17.7583, -12.8172) (17.7692, -12.8248) (17.7802, -12.8325) (17.7913, -12.8401) (17.8023, -12.8477) (17.8112, -12.8539) (17.8179, -12.8584) (17.8224, -12.8615) (17.8246, -12.863) knots 0 0 0 0 0 0 0.00416667 0.00833333 0.0125 0.01666667 0.02083333 0.025 0.02916667 0.03333333 0.0375 0.04166667 0.04583333 0.05 0.05416667 0.05833333 0.0625 0.06666667 0.07083333 0.075 0.07916667 0.08333333 0.0875 0.09166667 0.09583333 0.1 0.10416667 0.10833333 0.1125 0.11666667 0.12083333 0.125 0.12916667 0.13333333 0.1375 0.14166667 0.14583333 0.15 0.15416667 0.15833333 0.1625 0.16666667 0.17083333 0.175 0.17916667 0.18333333 0.1875 0.19166667 0.19583333 0.2 0.20416667 0.20833333 0.2125 0.21666667 0.22083333 0.225 0.22916667 0.23333333 0.2375 0.24166667 0.24583333 0.25 0.25416667 0.25833333 0.2625 0.26666667 0.27083333 0.275 0.27916667 0.28333333 0.2875 0.29166667 0.29583333 0.3 0.30416667 0.30833333 0.3125 0.31666667 0.32083333 0.325 0.32916667 0.33333333 0.3375 0.34166667 0.34583333 0.35 0.35416667 0.35833333 0.3625 0.36666667 0.37083333 0.375 0.37916667 0.38333333 0.3875 0.39166667 0.39583333 0.4 0.40416667 0.40833333 0.4125 0.41666667 0.42083333 0.425 0.42916667 0.43333333 0.4375 0.44166667 0.44583333 0.45 0.45416667 0.45833333 0.4625 0.46666667 0.47083333 0.475 0.47916667 0.48333333 0.4875 0.49166667 0.49583333 0.5 0.50416667 0.50833333 0.5125 0.51666667 0.52083333 0.525 0.52916667 0.53333333 0.5375 0.54166667 0.54583333 0.55 0.55416667 0.55833333 0.5625 0.56666667 0.57083333 0.575 0.57916667 0.58333333 0.5875 0.59166667 0.59583333 0.6 0.60416667 0.60833333 0.6125 0.61666667 0.62083333 0.625 0.62916667 0.63333333 0.6375 0.64166667 0.64583333 0.65 0.65416667 0.65833333 0.6625 0.66666667 0.67083333 0.675 0.67916667 0.68333333 0.6875 0.69166667 0.69583333 0.7 0.70416667 0.70833333 0.7125 0.71666667 0.72083333 0.725 0.72916667 0.73333333 0.7375 0.74166667 0.74583333 0.75 0.75416667 0.75833333 0.7625 0.76666667 0.77083333 0.775 0.77916667 0.78333333 0.7875 0.79166667 0.79583333 0.8 0.80416667 0.80833333 0.8125 0.81666667 0.82083333 0.825 0.82916667 0.83333333 0.8375 0.84166667 0.84583333 0.85 0.85416667 0.85833333 0.8625 0.86666667 0.87083333 0.875 0.87916667 0.88333333 0.8875 0.89166667 0.89583333 0.9 0.90416667 0.90833333 0.9125 0.91666667 0.92083333 0.925 0.92916667 0.93333333 0.9375 0.94166667 0.94583333 0.95 0.95416667 0.95833333 0.9625 0.96666667 0.97083333 0.975 0.97916667 0.98333333 0.9875 0.99166667 0.99583333 1 1 1 1 1 1
  arc A81 (22.7084, -8.6029) -> (23.3609, -7.8781) centre (0, 12.5) ccw
  line L152 (20.9569, 32.6094) -> (20.7445, 32.4055)
  line L153 (22.9441, 30.3086) -> (22.7115, 30.1281)
  line L154 (22.1898, 31.2401) -> (22.1904, 31.2406)